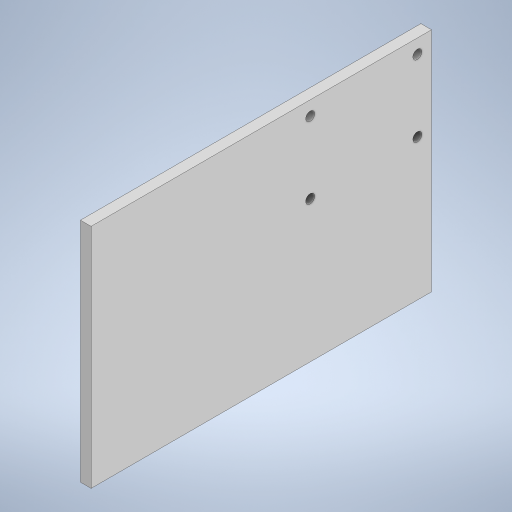
# Autodesk Inventor part: base plate
Saved by Autodesk Inventor 2024.2 (Build 282272000, 272)
## iProperties
Created: 2024-08-06
Part Number: base plate
Material: Generic
Document SubType Name: Modeling
Designer: Tom
Density: 1 g/cm^3
Appearance: Default
Author: Tom
Autodesk Inventor part; units mm, degrees
ref_plane "YZ Plane" through (0, 0, 0) normal (1, 0, 0) x (0, 1, 0)
ref_plane "XZ Plane" through (0, 0, 0) normal (0, 1, 0) x (-1, 0, 0)
ref_plane "XY Plane" through (0, 0, 0) normal (0, 0, 1) x (1, 0, 0)
sketch "Sketch1" plane through (0, 0, 0) normal (1, 0, 0) x (0, 1, 0)
  line L0 (0, 0) -> (101.6, 0)
  line L1 (101.6, 0) -> (101.6, -152.4)
  line L2 (101.6, -152.4) -> (0, -152.4)
  line L3 (0, -152.4) -> (0, 0)
  dimension "d0" = 101.6
  dimension "d1" = 152.4
  constraints: 8 end point, 2 parallel, 1 horizontal, 1 perpendicular
  measures "d0" distance of L0.start L0.end
  measures "d1" distance of L0.end L1.end
extrude "Extrusion1" add sketch "Sketch1" along normal blind 4.7625
sketch "Sketch3" plane through (4.7625, 0, 0) normal (1, 0, 0) x (0, 0, -1)
  circle A0 centre (146.05, 63.246) radius 1.9939
  circle A1 centre (146.05, 95.25) radius 1.9939
  line L0 (152.4, 0) -> (152.4, 101.6) projected
  line L1 (152.4, 101.6) -> (0, 101.6) projected
  point P0 (0, 0)
  dimension "d4" = 32.004
  dimension "d5" = 3.9878
  dimension "d6" = 3.9878
  dimension "d7" = 6.35
  dimension "d8" = 6.35
  dimension "d12" = 6.35
  constraints: 2 centre point
  measures "d4" distance of A1.centre A0.centre
  measures "d5" diameter of A1
  measures "d6" diameter of A0
  measures "d7" distance from line of L0 A1.centre
  measures "d8" distance from line of L1 A1.centre
  measures "d12" distance from line of L0 A0.centre
extrude "Extrusion2" cut sketch "Sketch3" against normal through all
sketch "Sketch4" plane through (4.7625, 0, 0) normal (1, 0, 0) x (0, 0, -1)
  circle A0 centre (98.0694, 95.25) radius 1.9939
  circle A1 centre (98.0694, 63.246) radius 1.9939
  circle A2 centre (146.05, 95.25) radius 1.9939 projected
  circle A3 centre (146.05, 63.246) radius 1.9939 projected
  point P0 (0, 0)
  dimension "d13" = 47.9806
  dimension "d14" = 47.9806
  dimension "d15" = 3.9878
  dimension "d16" = 3.9878
  constraints: 2 centre point
  measures "d13" distance of A2.centre A0.centre
  measures "d14" distance of A3.centre A1.centre
  measures "d15" diameter of A0
  measures "d16" diameter of A1
extrude "Extrusion3" cut sketch "Sketch4" against normal through all contours A0 | A1
body "Solid1"
